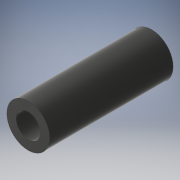
# Autodesk Inventor part: fc17_009
Saved by Autodesk Inventor 2017.1 (Build 211199000, 199)
## iProperties
Category: Micellaneous
Company: Autodesk Inc.
Created: 2016-12-14
Part Number: fc17_009
Material: ABS Plastic
Document SubType Name: Modeling
Designer: Autodesk Inc.
Density: 1.06 g/cm^3
Appearance: Smooth - Black
Catalog Web Link: http://www.andymark.com/product-p/am-0755.htm
Vendor: AndyMark Inc.
Author: Autodesk Inc.
Keywords: FIRST Choice
Autodesk Inventor part; units mm, degrees
ref_plane "YZ Plane" through (0, 0, 0) normal (1, 0, 0) x (0, 1, 0)
ref_plane "XZ Plane" through (0, 0, 0) normal (0, 1, 0) x (-1, 0, 0)
ref_plane "XY Plane" through (0, 0, 0) normal (0, 0, 1) x (1, 0, 0)
sketch "Sketch1" plane through (0, 0, 0) normal (0, 1, 0) x (-1, 0, 0)
  circle A0 centre (0, 0) radius 8.509
  circle A1 centre (0, 0) radius 4.826
  dimension "d0" = 17.018
  dimension "d1" = 9.652
  constraints: 2 centre point, 2 coincident
  measures "d0" diameter of A0
  measures "d1" diameter of A1
extrude "Extrusion1" add sketch "Sketch1" against normal blind 49.276
body "Solid1"
